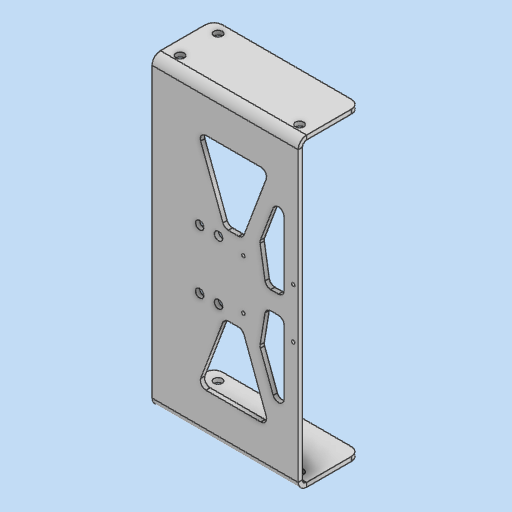
# Autodesk Inventor part: NeckMiddleBracket
Saved by Autodesk Inventor 2025.2 (Build 292293000, 293)
## iProperties
Created: 2025-09-15
Part Number: NeckMiddleBracket
Material: Generic
Document SubType Name: Sheet Metal
Designer: valer
Density: 1 g/cm^3
Sheet Metal Rule: Default
Appearance: Default
Author: valer
Autodesk Inventor part; units mm, degrees
ref_plane "YZ Plane" through (0, 0, 0) normal (1, 0, 0) x (0, 1, 0)
ref_plane "XZ Plane" through (0, 0, 0) normal (0, 1, 0) x (-1, 0, 0)
ref_plane "XY Plane" through (0, 0, 0) normal (0, 0, 1) x (1, 0, 0)
sketch "Base" plane through (0, 0, 0) normal (0, 0, 1) x (1, 0, 0)
  line L0 (-128.0777, -108.501) -> (-24.0777, -108.501)
  line L1 (-24.0777, -108.501) -> (-24.0777, 108.549)
  line L2 (-24.0777, 108.549) -> (-128.0777, 108.549)
  line L3 (-128.0777, 108.549) -> (-128.0777, -108.501)
  line L4 (-122.0777, -108.501) -> (-44.6445, -108.501) construction
  line L5 (-122.0777, 108.549) -> (-44.6445, 108.549) construction
  line L6 (-36.0777, -111.549) -> (-30.0777, -111.549) construction
  point P0 (0, 0)
  dimension "d0" = 6
  measures "d0" distance from line of L1 L6.end
extrude "Plate1" add sketch "Base" along normal blind 3
sketch "Sketch2" plane through (-128.0777, -105.501, 3) normal (0, -1, 0) x (1, 0, 0)
  line L0 (104, 0) -> (0, 0)
  line L1 (0, 0) -> (0, -44)
  line L2 (0, -44) -> (104, -44)
  line L3 (104, -44) -> (104, 0)
  constraints: 6 end point, 1 horizontal, 1 perpendicular, 1 vertical
edge flange "FlangeFeature" height 44 angle 90 thickness 3 bend radius 3 thickness toward (0, -1, 0) relief straight relief width 3 relief depth 1.5 corner gap 3 corner form 0 edges at (-76.0777, -108.501, 0) (-76.0777, 108.549, 0) wall of the first edge with corners at (-24.0777, -105.501, 3) (-128.0777, -105.501, 3) (-128.0777, -105.501, -41) (-24.0777, -105.501, -41)
bend "Bend1"
corner "Corner1"
sketch "VentHoles" plane through (0, 0, 3) normal (0, 0, 1) x (1, 0, 0)
  line L0 (-24.0777, -102.501) -> (-128.0777, -102.501) construction
  line L1 (-128.0777, 102.549) -> (-24.0777, 102.549) construction
  line L2 (-24.0777, 0.024) -> (-128.0777, 0.024) construction
  line L3 (-128.0777, 102.549) -> (-128.0777, -102.501) construction
  line L4 (-118.0777, 78.501) -> (-106.0777, 78.501)
  line L5 (-24.0777, 102.549) -> (-24.0777, -102.501) construction
  line L6 (-76.6193, -27.976) -> (-95.4673, -78.501)
  line L7 (-95.4673, -78.501) -> (-44.7509, -78.501)
  line L8 (-44.7509, -78.501) -> (-63.5988, -27.976)
  line L9 (-63.5988, -27.976) -> (-76.6193, -27.976)
  line L10 (-51.3194, -32.2818) -> (-47.0982, -6.4928)
  line L11 (-47.0982, -6.4928) -> (-34.0777, -6.4928)
  line L12 (-34.0777, -6.4928) -> (-34.0777, -78.501)
  line L13 (-34.0777, -78.501) -> (-51.3194, -32.2818)
  line L14 (-44.7509, -78.501) -> (-34.0777, -78.501) construction
  line L15 (-76.6193, 28.024) -> (-95.4673, 78.549)
  line L16 (-95.4673, 78.549) -> (-44.7509, 78.549)
  line L17 (-44.7509, 78.549) -> (-63.5988, 28.024)
  line L18 (-63.5988, 28.024) -> (-76.6193, 28.024)
  line L19 (-51.3194, 32.3298) -> (-47.0982, 6.5408)
  line L20 (-47.0982, 6.5408) -> (-34.0777, 6.5408)
  line L21 (-34.0777, 6.5408) -> (-34.0777, 78.549)
  line L22 (-34.0777, 78.549) -> (-51.3194, 32.3298)
  point P0 (0, 0)
  dimension "d24" = 69.542
  dimension "d25" = 69.542
  dimension "d26" = 10
  dimension "d28" = 10
  dimension "d32" = 6.5168
  dimension "d60" = 28
  dimension "d61" = 24
  dimension "d62" = 50.7164
  dimension "d63" = 99.296
  dimension "d64" = 25.789
  constraints: 38 end point, 8 symmetric about line, 4 parallel, 3 horizontal, 2 midpoint
  measures "d24" angle of L6 L7
  measures "d25" angle of L8 L7
  measures "d26" distance between parallel lines of L5 L12
  measures "d28" distance between parallel lines of L13 L8
  measures "d32" distance between parallel lines of L2 L11
  measures "d60" distance between parallel lines of L2 L9
  measures "d61" distance between parallel lines of L7 L0
  measures "d62" distance of L6.end L7.end
  measures "d63" angle of L11 L10
  measures "d64" vertical distance of L10.start L10.end
extrude "VentHolesFeature" cut sketch "VentHoles" against normal blind 3
fillet "InsideFilletsFeature" radius 4 16 edges at (-95.4673, -78.501, 1.5) (-44.7509, -78.501, 1.5) (-63.5988, -27.976, 1.5) (-76.6193, -27.976, 1.5) (-95.4673, 78.549, 1.5) (-76.6193, 28.024, 1.5) (-63.5988, 28.024, 1.5) (-44.7509, 78.549, 1.5) (-51.3194, 32.3298, 1.5) (-47.0982, 6.5408, 1.5) (-34.0777, 6.5408, 1.5) (-34.0777, 78.549, 1.5) (-34.0777, -78.501, 1.5) (-51.3194, -32.2818, 1.5) (-47.0982, -6.4928, 1.5) (-34.0777, -6.4928, 1.5)
sketch "NeckMountHoles" plane through (0, 0, 3) normal (0, 0, 1) x (1, 0, 0)
  circle A0 centre (-94.1014, -21) radius 2.7 projected
  circle A1 centre (-80.7014, -21) radius 2.7 projected
  circle A2 centre (-94.1014, 21) radius 2.7 projected
  circle A3 centre (-80.7014, 21) radius 2.7 projected
  point P0 (0, 0)
hole "NeckMountHolesFeature" at (-94.1014, -21, 3) at (-80.7014, -21, 3) at (-80.7014, 21, 3) at (-94.1014, 21, 3) direction (0, 0, -1) diameter 6 depth 3 tip angle 118
sketch "SideHoles" plane through (-128.0777, -105.501, -41) normal (0, 1, 0) x (1, 0, 0)
  circle A0 centre (10, -34) radius 3 projected
  circle A1 centre (10, -7) radius 3 projected
  circle A2 centre (95, -34) radius 3 projected
  point P0 (128.0777, -41)
extrude "SideHolesFeature" cut sketch "SideHoles" along normal through all both and the other way through all
fillet "FlangeFilletsFeature" radius 6 4 edges at (-128.0777, -107.001, -41) (-24.0777, -107.001, -41) (-128.0777, 107.049, -41) (-24.0777, 107.049, -41)
sketch "TiltDriverMountHoles" plane through (0, 0, 3) normal (0, 0, 1) x (1, 0, 0)
  circle A0 centre (-63.0777, -17.75) radius 1.6 construction
  circle A1 centre (-63.0777, 17.75) radius 1.6 construction
  circle A2 centre (-27.5777, 17.75) radius 1.6 construction
  circle A3 centre (-27.5777, -17.75) radius 1.6 construction
  circle A4 centre (-63.0777, -17.75) radius 1.2
  circle A5 centre (-63.0777, 17.75) radius 1.2
  circle A6 centre (-27.5777, -17.75) radius 1.2
  circle A7 centre (-27.5777, 17.75) radius 1.2
  point P0 (0, 0)
  dimension "d65" = 2.4
  constraints: 4 centre point, 4 coincident, 3 equal radius
  measures "d65" diameter of A4
extrude "TiltDriverMountHolesFeature" cut sketch "TiltDriverMountHoles" against normal through all
equation "\"d25\" = d24"
equation "\"d26\" = d17"
equation "\"d28\" = d17"
equation "\"d32\" = 0.5 * d29"
equation "\"d34\" = Thickness"
equation "\"d55\" = Thickness"
equation "\"d57\" = Thickness"
equation "\"d66\" = Thickness"
equation "\"d1\" = Thickness"
equation "\"d2\" = BendReliefWidth"
equation "\"d3\" = BendReliefDepth"
equation "\"d4\" = MinimumRemnant"
equation "\"d5\" = TransitionRadius"
equation "\"d8\" = BendRadius"
equation "\"d9\" = CornerReliefSize"
equation "\"d10\" = GapSize"
equation "\"d11\" = JacobiRadiusSize"
equation "\"BendRadius\" = Thickness"
equation "\"BendReliefWidth\" = Thickness"
equation "\"BendReliefDepth\" = 0.5 * Thickness"
equation "\"CornerReliefSize\" = 4 * Thickness"
equation "\"MinimumRemnant\" = 2 * Thickness"
equation "\"TransitionRadius\" = BendRadius"
equation "\"JacobiRadiusSize\" = BendRadius"
equation "\"GapSize\" = Thickness"
equation "\"d17\" = 10"
equation "\"d29\" = 13.033682"
equation "\"Thickness\" = 3"
body "Solid1"
